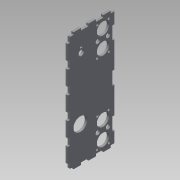
# Autodesk Inventor part: srf kiri
Saved by Autodesk Inventor 2015 SP1 (Build 190203100, 203)
## iProperties
Created: 2015-02-15
Part Number: srf kiri
Material: Generic
Document SubType Name: Modeling
Designer: Rafi Kurnia Putra
Density: 1 g/cm^3
Appearance: Default
Author: Rafi Kurnia Putra
Autodesk Inventor part; units mm, degrees
ref_plane "YZ Plane" through (0, 0, 0) normal (1, 0, 0) x (0, 1, 0)
ref_plane "XZ Plane" through (0, 0, 0) normal (0, 1, 0) x (-1, 0, 0)
ref_plane "XY Plane" through (0, 0, 0) normal (0, 0, 1) x (1, 0, 0)
sketch "Sketch1" plane through (0, 0, 0) normal (1, 0, 0) x (0, 1, 0)
  line L0 (63, -58.6109) -> (63.0005, -43.5826)
  line L1 (60.0005, -43.5825) -> (63.0005, -43.5826)
  line L2 (60.0011, -26.0825) -> (60.0005, -43.5825)
  line L3 (63.0011, -26.0826) -> (60.0011, -26.0825)
  line L4 (63.0011, -26.0826) -> (63.0018, -7.1898)
  line L5 (63.0018, -7.1898) -> (63.0023, 9.6674)
  line L6 (60, 9.6674) -> (63.0023, 9.6674)
  line L7 (60, 27.1674) -> (60, 9.6674)
  line L8 (63, 27.1674) -> (60, 27.1674)
  line L9 (63, 27.1674) -> (63, 44.0245)
  line L10 (63, 44.0245) -> (63, 62.6674)
  line L11 (60, 62.6674) -> (63, 62.6674)
  line L12 (60, 80.1674) -> (60, 62.6674)
  line L13 (63, 80.1674) -> (60, 80.1674)
  line L14 (63, 80.1674) -> (63, 95.2386)
  circle A0 centre (18.25, 69.1244) radius 3.75
  line L15 (16.75, 76.1244) -> (16.75, 75.1244)
  line L16 (17.25, 74.6244) -> (19.25, 74.6244)
  arc A1 (19.25, 74.6244) -> (19.75, 75.1244) centre (19.25, 75.1244) ccw
  line L17 (19.75, 75.1244) -> (19.75, 76.1244)
  arc A2 (19.75, 76.1244) -> (19.25, 76.6244) centre (19.25, 76.1244) ccw
  line L18 (19.25, 76.6244) -> (17.25, 76.6244)
  arc A3 (17.25, 76.6244) -> (16.75, 76.1244) centre (17.25, 76.1244) ccw
  arc A4 (16.75, 75.1244) -> (17.25, 74.6244) centre (17.25, 75.1244) ccw
  circle A5 centre (55.3, -15.9142) radius 1.5875
  circle A6 centre (54.4, -35.289) radius 2.95
  circle A7 centre (47.5, -23.5892) radius 8.25
  circle A8 centre (47.5, -46.9892) radius 8.25
  circle A9 centre (39.7, -54.6642) radius 1.5875
  circle A10 centre (40.6, -35.289) radius 2.95
  circle A11 centre (40.0677, -15.9142) radius 1.5875
  circle A12 centre (55.6677, -54.6642) radius 1.5875
  line L19 (55.3, -15.9142) -> (39.7, -54.6642) construction
  line L20 (55.6677, -54.6642) -> (40.0677, -15.9142) construction
  circle A13 centre (16.9008, -13.4535) radius 9.2
  circle A14 centre (55.3, 90.5858) radius 1.5875
  circle A15 centre (40.0677, 90.5858) radius 1.5875
  circle A16 centre (47.5, 82.9108) radius 8.25
  circle A17 centre (54.4, 71.211) radius 2.95
  circle A18 centre (40.6, 71.211) radius 2.95
  circle A19 centre (47.5, 59.5108) radius 8.25
  circle A20 centre (39.7, 51.8358) radius 1.5875
  circle A21 centre (55.6677, 51.8358) radius 1.5875
  line L21 (55.3, 90.5858) -> (39.7, 51.8358) construction
  line L22 (55.6677, 51.8358) -> (40.0677, 90.5858) construction
  line L23 (3, 8.4171) -> (0, 8.4171)
  line L24 (0, 8.4171) -> (0, 28.4171)
  line L25 (0, 28.4171) -> (3, 28.4171)
  line L26 (3, 28.4171) -> (3, 8.4171) construction
  line L27 (3, 8.4171) -> (0, 28.4171) construction
  line L28 (0, 8.4171) -> (3, 28.4171) construction
  line L29 (31.5, 18.3138) -> (31.5, 31.364) construction
  line L30 (31.5, 18.3138) -> (40.6, 18.3138) construction
  line L31 (3, -21.5829) -> (0, -21.5829)
  line L32 (0, -21.5829) -> (0, -1.5829)
  line L33 (0, -1.5829) -> (3, -1.5829)
  line L34 (3, -51.5829) -> (0, -51.5829)
  line L35 (0, -51.5829) -> (0, -31.5829)
  line L36 (0, -31.5829) -> (3, -31.5829)
  line L37 (3, 38.4171) -> (0, 38.4171)
  line L38 (0, 38.4171) -> (0, 58.4171)
  line L39 (0, 58.4171) -> (3, 58.4171)
  line L40 (3, 8.4171) -> (0, 8.4171)
  line L41 (0, 8.4171) -> (0, 28.4171)
  line L42 (0, 28.4171) -> (3, 28.4171)
  line L43 (3, -21.5829) -> (0, -21.5829)
  line L44 (0, -21.5829) -> (0, -1.5829)
  line L45 (0, -1.5829) -> (3, -1.5829)
  line L46 (3, 68.4171) -> (0, 68.4171)
  line L47 (0, 68.4171) -> (0, 88.4171)
  line L48 (0, 88.4171) -> (3, 88.4171)
  line L49 (3, 38.4171) -> (0, 38.4171)
  line L50 (0, 38.4171) -> (0, 58.4171)
  line L51 (0, 58.4171) -> (3, 58.4171)
  line L52 (3, 8.4171) -> (0, 8.4171)
  line L53 (0, 8.4171) -> (0, 28.4171)
  line L54 (0, 28.4171) -> (3, 28.4171)
  line L55 (3, -51.5829) -> (3, -58.6109)
  line L56 (3, -31.5829) -> (3, -21.5829)
  line L57 (3, -1.5829) -> (3, 8.4171)
  line L58 (3, 28.4171) -> (3, 38.4171)
  line L59 (3, 58.4171) -> (3, 68.4171)
  line L60 (3, 88.4171) -> (3, 95.2386)
  line L61 (28, -58.6109) -> (28, -61.6109)
  line L62 (28, -61.6109) -> (38, -61.6109)
  line L63 (38, -61.6109) -> (38, -58.6109)
  line L64 (38, -58.6109) -> (28, -61.6109) construction
  line L65 (28, -58.6109) -> (38, -61.6109) construction
  line L66 (48, -58.6109) -> (48, -61.6109)
  line L67 (48, -61.6109) -> (58, -61.6109)
  line L68 (58, -61.6109) -> (58, -58.6109)
  line L69 (58, -58.6109) -> (48, -61.6109) construction
  line L70 (48, -58.6109) -> (58, -61.6109) construction
  line L71 (8, -58.6109) -> (8, -61.6109)
  line L72 (8, -61.6109) -> (18, -61.6109)
  line L73 (18, -61.6109) -> (18, -58.6109)
  line L74 (18, -58.6109) -> (8, -61.6109) construction
  line L75 (8, -58.6109) -> (18, -61.6109) construction
  line L76 (28, -58.6109) -> (28, -61.6109)
  line L77 (28, -61.6109) -> (38, -61.6109)
  line L78 (38, -61.6109) -> (38, -58.6109)
  line L79 (38, -58.6109) -> (28, -61.6109) construction
  line L80 (28, -58.6109) -> (38, -61.6109) construction
  line L81 (63, -58.6109) -> (58, -58.6109)
  line L82 (48, -58.6109) -> (38, -58.6109)
  line L83 (28, -58.6109) -> (18, -58.6109)
  line L84 (8, -58.6109) -> (3, -58.6109)
  line L85 (28, 95.2386) -> (28, 98.2386)
  line L86 (28, 98.2386) -> (38, 98.2386)
  line L87 (38, 98.2386) -> (38, 95.2386)
  line L88 (38, 95.2386) -> (28, 98.2386) construction
  line L89 (28, 95.2386) -> (38, 98.2386) construction
  line L90 (58, 98.2386) -> (58, 95.2386)
  line L91 (48, 98.2386) -> (58, 98.2386)
  line L92 (58, 95.2386) -> (48, 98.2386) construction
  line L93 (48, 95.2386) -> (58, 98.2386) construction
  line L94 (48, 95.2386) -> (48, 98.2386)
  line L95 (18, 98.2386) -> (18, 95.2386)
  line L96 (8, 98.2386) -> (18, 98.2386)
  line L97 (18, 95.2386) -> (8, 98.2386) construction
  line L98 (8, 95.2386) -> (18, 98.2386) construction
  line L99 (8, 95.2386) -> (8, 98.2386)
  line L100 (38, 98.2386) -> (38, 95.2386)
  line L101 (28, 98.2386) -> (38, 98.2386)
  line L102 (38, 95.2386) -> (28, 98.2386) construction
  line L103 (28, 95.2386) -> (38, 98.2386) construction
  line L104 (28, 95.2386) -> (28, 98.2386)
  line L105 (48, 95.2386) -> (38, 95.2386)
  line L106 (28, 95.2386) -> (18, 95.2386)
  line L107 (58, 95.2386) -> (63, 95.2386)
  line L108 (8, 95.2386) -> (3, 95.2386)
  point P0 (0, 0)
  point P1 (47.6838, -34.8326)
  point P2 (47.6838, -34.8326)
  point P3 (47.6838, -34.8326)
  point P4 (47.6838, 71.6674)
  point P5 (47.6838, 71.6674)
  point P6 (47.6838, 71.6674)
  point P7 (47.6838, 71.6674)
  point P8 (1.5, 18.4171)
  point P9 (60, 18.4174)
  point P10 (33, -60.1109)
  point P11 (53, -60.1109)
  point P12 (13, -60.1109)
  point P13 (33, -60.1109)
  point P14 (33, 96.7386)
  point P15 (53, 96.7386)
  point P16 (13, 96.7386)
  point P17 (33, 96.7386)
  dimension "d0" = 7.8
  dimension "d1" = 7.8
  dimension "d2" = 7.8
  dimension "d3" = 7.8
  dimension "d7" = 3
  dimension "d8" = 20
  dimension "d11" = 30
  dimension "d14" = 30
  dimension "d17" = 10
  dimension "d18" = 3
  dimension "d21" = 20
  dimension "d24" = 20
  constraints: 218 end point, 22 centre point, 20 symmetric about line, 19 midpoint, 8 point on circle, 7 collinear, 6 horizontal, 5 point on line, 4 vertical, 3 parallel, 2 coincident, 1 perpendicular, 86 other
  measures "d0" horizontal distance of L19.end A8.centre
  measures "d1" horizontal distance of A7.centre L19.start
  measures "d2" horizontal distance of L21.end A19.centre
  measures "d3" horizontal distance of A16.centre L21.start
  measures "d7" distance of L24.end L25.end
  measures "d8" distance of L23.end L24.end
  measures "d11" distance of L23.start L31.start
  measures "d14" distance of L23.start L37.start
  measures "d17" distance of L62.end L61.end
  measures "d18" distance of L61.end L61.start
  measures "d21" distance of L63.end L68.end
  measures "d24" distance of L63.end L73.end
extrude "Extrusion1" add sketch "Sketch1" along normal blind 3
body "Solid1"
